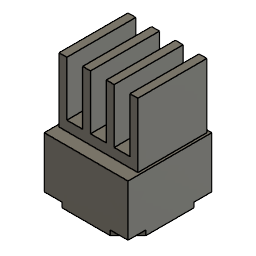
Camera Module (Autodesk Fusion 360 design; units mm, degrees)
part number: 2026-08-01-18-53-29-409
Autodesk Fusion 360 part; units mm, degrees
note: some values were not read from the file. Set by a fixed rule: which sketch regions a step uses.
sketch "Sketch1" plane through (0, 0, 0) normal (0, 1, 0) x (1, 0, 0)
  line L0 (0, 0) -> (8.5, 0)
  line L1 (8.5, 0) -> (8.5, 8.5)
  line L2 (8.5, 8.5) -> (0, 8.5)
  line L3 (0, 8.5) -> (0, 0)
  dimension "d1" = 8.5
  dimension "d2" = 8.5
  constraint horizontal L0
  constraint vertical L1
  constraint horizontal L2
  constraint vertical L3
  constraint coincident L0.start L3.end
  measures "d1" distance of L0.start L0.end
  measures "d2" distance of L0.start L2.end
extrude "Extrude1" add sketch "Sketch1" along normal blind 5.2
sketch "Sketch2" plane through (0, 5.2, 0) normal (0, 1, 0) x (-1, 0, 0)
  line L0 (0, -8.5) -> (0, 0)
  line L1 (0, 0) -> (-8.5, 0)
  line L2 (-8.5, 0) -> (-8.5, -8.5)
  line L3 (-8.5, -8.5) -> (0, -8.5)
  line L4 (-0.25, -8.25) -> (-8.25, -8.25)
  line L5 (-8.25, -8.25) -> (-8.25, -1.25)
  line L6 (-8.25, -1.25) -> (-0.25, -1.25)
  line L7 (-0.25, -1.25) -> (-0.25, -8.25)
  dimension "d5" = 8
  dimension "d6" = 7
  dimension "d7" = 0.25
  dimension "d8" = 0.25
  constraint horizontal L4
  constraint vertical L5
  constraint horizontal L6
  constraint vertical L7
  measures "d5" distance of L4.start L4.end
  measures "d6" distance of L4.start L6.end
  measures "d7" distance of L2 L5
  measures "d8" distance of L3 L4
sketch "Sketch3" plane through (0, 5.2, 0) normal (0, 1, 0) x (-1, 0, 0)
extrude "Extrude2" add sketch "Sketch2" along normal blind 1 contours L4 L5 L6 L7
sketch "Sketch4" plane through (0, 6.2, 0) normal (0, 1, 0) x (-1, 0, 0)
  line L0 (-0.25, -1.25) -> (-8.25, -1.25)
  line L1 (-8.25, -1.25) -> (-8.25, -8.25)
  line L2 (-8.25, -8.25) -> (-0.25, -8.25)
  line L3 (-0.25, -8.25) -> (-0.25, -1.25)
  line L4 (-0.25, -8.25) -> (-1.05, -8.25)
  line L5 (-1.05, -8.25) -> (-1.05, -1.25)
  line L6 (-1.05, -1.25) -> (-0.25, -1.25)
  line L7 (-0.25, -1.25) -> (-0.25, -8.25)
  line L8 (-2.65, -8.25) -> (-3.45, -8.25)
  line L9 (-2.65, -1.25) -> (-2.65, -8.25)
  line L10 (-3.45, -8.25) -> (-3.45, -1.25)
  line L11 (-3.45, -1.25) -> (-2.65, -1.25)
  line L12 (-5.05, -8.25) -> (-5.85, -8.25)
  line L13 (-5.05, -1.25) -> (-5.05, -8.25)
  line L14 (-5.85, -8.25) -> (-5.85, -1.25)
  line L15 (-5.85, -1.25) -> (-5.05, -1.25)
  line L16 (-7.45, -8.25) -> (-8.25, -8.25)
  line L17 (-7.45, -1.25) -> (-7.45, -8.25)
  line L18 (-8.25, -8.25) -> (-8.25, -1.25)
  line L19 (-8.25, -1.25) -> (-7.45, -1.25)
  dimension "d11" = 0.8
  dimension "d12" = 7
  dimension "d15" = -7.2
  dimension "d16" = 0
  constraint horizontal L4
  constraint vertical L5
  constraint horizontal L6
  constraint vertical L7
  constraint coincident L2.end L3.start
  measures "d11" distance of L2.end L4.end
  measures "d12" distance of L2.end L0.start
extrude "Extrude3" add sketch "Sketch4" along normal blind 5.519 contours L0 L2 L3 L4 L5 L6 L7 | L0 L2 L8 L9 L10 L11 | L0 L2 L12 L13 L14 L15 | L0 L1 L2 L16 L17 L18 L19
sketch "Sketch5" plane through (0, 0, 0) normal (0, -1, 0) x (1, 0, 0)
  line L0 (0, 0) -> (0, -8.5)
  line L1 (0, -8.5) -> (8.5, -8.5)
  line L2 (8.5, -8.5) -> (8.5, 0)
  line L3 (8.5, 0) -> (0, 0)
  line L4 (6.7, -8.5) -> (1.8, -8.5)
  line L5 (0, -6.7) -> (0, -1.8)
  line L6 (1.8, 0) -> (6.7, 0)
  line L7 (8.5, -1.8) -> (8.5, -6.7)
  line L8 (0, -1.8) -> (1.8, 0)
  line L9 (6.7, 0) -> (8.5, -1.8)
  line L10 (1.8, -8.5) -> (0, -6.7)
  line L11 (6.7, -8.5) -> (8.5, -6.7)
  point P0 (8.5, -8.5)
  point P1 (0, -8.5)
  point P2 (8.5, 0)
  dimension "d19" = 8.5
  dimension "d20" = 8.5
  dimension "d23" = 1.8
  dimension "d24" = 1.8
  dimension "d25" = 1.8
  dimension "d26" = 1.8
  dimension "d27" = 1.8
  dimension "d28" = 1.8
  dimension "d29" = 1.8
  dimension "d30" = 1.8
  constraint horizontal L4
  constraint vertical L5
  constraint horizontal L6
  constraint vertical L7
  constraint coincident L0.start L5
  constraint coincident L0.start L6
  constraint coincident L2 L7
  constraint coincident P2 L6
  constraint coincident P2 L7
  constraint coincident P1 L4
  constraint coincident P1 L5
  constraint coincident P0 L4
  constraint coincident P0 L7
  measures "d19" distance of P0 P1
  measures "d20" distance of P1 L0.start
  measures "d23" distance of L0.start L5.end
  measures "d24" distance of L0.start L6.start
  measures "d25" distance of P2 L6.end
  measures "d26" distance of P2 L7.start
  measures "d27" distance of P1 L4.end
  measures "d28" distance of P1 L5.start
  measures "d29" distance of P0 L4.start
  measures "d30" distance of P0 L7.end
extrude "Extrude4" add sketch "Sketch5" along normal blind 0.5 contours L0 L1 L2 L3 L4 L5 L6 L7 L8 L9 L10 L11
sketch "Sketch6" plane through (0, -0.5, 0) normal (0, -1, 0) x (1, 0, 0)
  line L0 (1.8, -8.5) -> (6.7, -8.5)
  line L1 (6.7, -8.5) -> (8.5, -6.7)
  line L2 (8.5, -6.7) -> (8.5, -1.8)
  line L3 (8.5, -1.8) -> (6.7, 0)
  line L4 (6.7, 0) -> (1.8, 0)
  line L5 (1.8, 0) -> (0, -1.8)
  line L6 (0, -1.8) -> (0, -6.7)
  line L7 (0, -6.7) -> (1.8, -8.5)
  circle A0 centre (4.25, -4.25) radius 3.35
  dimension "d32" = 6.7
  measures "d32" diameter of A0
extrude "Extrude5" cut sketch "Sketch6" against normal blind 0.346 contours A0
equation "d24 = d23"
